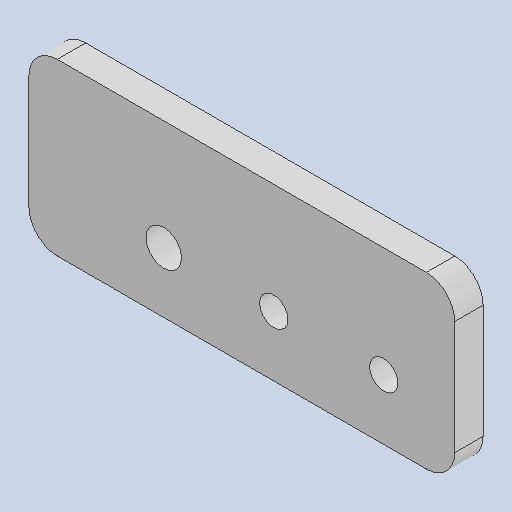
# Autodesk Inventor part: креп. пасс. ролика
Saved by Autodesk Inventor 2023.1 (Build 271208000, 208)
## iProperties
Created: 2025-12-01
Part Number: креп. пасс. ролика
Material: Типовые
Document SubType Name: Modeling
Designer: DELL
Density: 1 g/cm^3
Appearance: По умолчанию
Author: DELL
Autodesk Inventor part; units mm, degrees
ref_plane "YZ Plane" through (0, 0, 0) normal (1, 0, 0) x (0, 1, 0)
ref_plane "XZ Plane" through (0, 0, 0) normal (0, 1, 0) x (-1, 0, 0)
ref_plane "XY Plane" through (0, 0, 0) normal (0, 0, 1) x (1, 0, 0)
sketch "Эскиз1" plane through (0, 0, 0) normal (0, 0, 1) x (1, 0, 0)
  line L0 (20, -18.5) -> (20, -13.95) construction
  line L1 (-240, -18.5) -> (20, -18.5) construction
  line L2 (20, -18.5) -> (-40, -18.5)
  line L3 (-40, -18.5) -> (-40, 5.5)
  line L4 (-40, 5.5) -> (20, 5.5)
  line L5 (20, 5.5) -> (20, -18.5)
  point P0 (0, 0)
  dimension "d0" = 60
  dimension "d1" = 24
  constraints: 8 end point, 2 parallel, 1 horizontal, 1 perpendicular
  measures "d0" distance of L3.end L4.end
  measures "d1" distance of L2.end L3.end
extrude "Выдавливание1" add sketch "Эскиз1" along normal blind 4
fillet "Сопряжение1" radius 4 4 edges at (-40, 5.5, 2) (-40, -18.5, 2) (20, -18.5, 2) (20, 5.5, 2)
sketch "Эскиз2" plane through (0, 0, 4) normal (0, 0, 1) x (1, 0, 0)
  circle A0 centre (-21, 219) radius 7.5 construction
  line L0 (-21, 219) -> (-21, -6.68) construction
  arc A1 (-40, -14.5) -> (-36, -18.5) centre (-36, -14.5) ccw construction
  arc A2 (20, 1.5) -> (16, 5.5) centre (16, 1.5) ccw construction
  line L1 (-10, -6.5) -> (-40, -6.5) construction
  line L2 (-240, -6.68) -> (20, -6.68) construction
  line L3 (-240, -13.32) -> (20, -13.32) construction
  line L4 (-21, -6.68) -> (-21, -13.32) construction
  line L5 (-21, -13.32) -> (-21, -31) construction
  circle A3 centre (-21, -10) radius 2.5
  circle A4 centre (-5.5, -10) radius 2
  circle A5 centre (10, -10) radius 2
  line L6 (20, -14.5) -> (20, 1.5) projected
  point P0 (0, 0)
  dimension "d5" = 250
  dimension "d6" = 5
  dimension "d7" = 4
  dimension "d8" = 4
  dimension "d9" = 10
  dimension "d10" = 15.5
  constraints: 8 end point, 3 centre point, 3 vertical, 2 point on line, 1 horizontal, 1 midpoint
  measures "d5" distance of L0.start L5.end
  measures "d6" diameter of A3
  measures "d7" diameter of A4
  measures "d8" diameter of A5
  measures "d9" distance from line of L6 A5.centre
  measures "d10" distance of A4.centre A5.centre
extrude "Выдавливание2" cut sketch "Эскиз2" against normal blind 4
